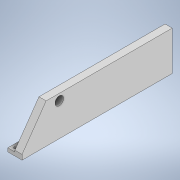
# Autodesk Inventor part: s_base4
Saved by Autodesk Inventor 2022 (Build 260153000, 153)
## iProperties
Created: 2021-08-20
Part Number: s_base4
Material: 一般
Document SubType Name: Modeling
Designer: yuta0
Density: 1 g/cm^3
Appearance: 既定
Author: yuta0
Autodesk Inventor part; units mm, degrees
ref_plane "YZ Plane" through (0, 0, 0) normal (1, 0, 0) x (0, 1, 0)
ref_plane "XZ Plane" through (0, 0, 0) normal (0, 1, 0) x (-1, 0, 0)
ref_plane "XY Plane" through (0, 0, 0) normal (0, 0, 1) x (1, 0, 0)
sketch "スケッチ1" plane through (0, 0, 0) normal (0, 0, 1) x (1, 0, 0)
  line L0 (-20, -2.5) -> (20, -2.5)
  line L1 (20, -2.5) -> (20, 2.5)
  line L2 (-20, 2.5) -> (-20, -2.5)
  line L3 (-20, -2.5) -> (20, 2.5) construction
  line L4 (20, -2.5) -> (-20, 2.5) construction
  line L5 (-10, 2.5) -> (10, 2.5)
  line L6 (10, 2.5) -> (10, 52.5)
  line L7 (10, 52.5) -> (-10, 52.5)
  line L8 (-10, 52.5) -> (-10, 2.5)
  line L9 (-10, 2.5) -> (10, 52.5) construction
  line L10 (10, 2.5) -> (-10, 52.5) construction
  line L11 (20, 2.5) -> (10, 2.5)
  line L12 (-10, 2.5) -> (-20, 2.5)
  line L13 (0, 52.5) -> (0, -2.5)
  point P0 (0, 0)
  point P1 (0, 27.5)
  point P2 (0, 27.5)
  point P3 (0, 0)
  dimension "d0" = 20
  dimension "d1" = 50
  dimension "d2" = 5
  dimension "d3" = 10
  constraints: 28 end point, 8 midpoint, 5 parallel, 2 horizontal, 2 perpendicular, 1 vertical alignment
  measures "d0" distance of L6.end L7.end
  measures "d1" distance of L5.end L6.end
  measures "d2" distance of L0.end L1.end
  measures "d3" distance between parallel lines of L8 L2
extrude "押し出し1" add sketch "スケッチ1" along normal mid plane 210 contours L2 L12 L5 L13 L0 | L5 L8 L7 L13
sketch "スケッチ8" plane through (-10, 2.5, 105) normal (-1, 0, 0) x (0, 0, 1)
  line L0 (-210, 50) -> (0, 50) projected
  line L1 (-33.61, 50) -> (0, 2)
  line L2 (0, -5) -> (0, 50) projected
  line L3 (-210, 0) -> (0, 0) projected
  point P0 (-105, -2.5)
  dimension "d60" = 2
  dimension "d68" = 145
  constraints: 2 end point, 2 point on line
  measures "d60" distance from line of L3 L1.end
  measures "d68" angle of L2 L1
extrude "押し出し5" cut sketch "スケッチ8" against normal blind 210
sketch "スケッチ9" plane through (-10, 2.5, -105) normal (-1, 0, 0) x (0, 0, 1)
  circle A0 centre (158, 41) radius 6.05
  line L0 (210, 2) -> (210, 0) projected
  line L1 (0, 0) -> (210, 0) projected
  point P0 (105, -2.5)
  dimension "d63" = 12.1
  dimension "d64" = 52
  dimension "d65" = 41
  constraints: 1 centre point
  measures "d63" diameter of A0
  measures "d64" distance from line of L0 A0.centre
  measures "d65" distance from line of L1 A0.centre
extrude "押し出し6" cut sketch "スケッチ9" against normal blind 210
sketch "スケッチ10" plane through (-20, 2.5, 105) normal (0, 1, 0) x (1, 0, 0)
  line L0 (0, 210) -> (0, 0) projected
  line L1 (10, 0) -> (0, 0) projected
  line L2 (0, 210) -> (10, 210) projected
  point P0 (20, 105)
  point P1 (5, 5)
  point P2 (5, 79.86)
  point P3 (5, 96.483)
  point P4 (5, 205)
  dimension "d69" = 5
  dimension "d70" = 5
  dimension "d71" = 74.86
  dimension "d72" = 16.623
  dimension "d73" = 5
  measures "d69" distance from line of L0 point (5, 5)
  measures "d70" distance from line of L1 point (5, 5)
  measures "d71" distance of point (5, 5) point (5, 79.86)
  measures "d72" distance of point (5, 79.86) point (5, 96.483)
  measures "d73" distance from line of L2 point (5, 205)
hole "穴5" at (-15, 2.5, -100) at (-15, 2.5, 100) direction (0, -1, 0) diameter 3.2 end through all
hole "穴6" at (-15, 2.5, 25.14) at (-15, 2.5, 8.517) direction (0, -1, 0) diameter 5.2 end through all
